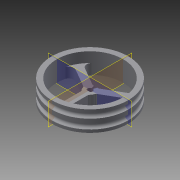
# Autodesk Inventor part: Rueda1
Saved by Autodesk Inventor 2013 (Build 170138000, 138)
## iProperties
Created: 2012-12-03
Part Number: Rueda1
Material: Generic
Document SubType Name: Modeling
Designer: ALUMNO
Density: 1 g/cm^3
Author: ALUMNO
Autodesk Inventor part; units mm, degrees
ref_plane "XY Plane" through (0, 0, 0) normal (0, 0, 1) x (1, 0, 0)
sketch "Sketch1" plane through (0, 0, 0) normal (0, 0, 1) x (1, 0, 0)
  line L0 (-19.5, 0) -> (19.5, 0) construction
  line L1 (-1.118, -1) -> (1.118, -1)
  line L2 (0, -3.5) -> (0, -10.5) construction
  line L3 (0, 31.6864) -> (0, -32.6182) construction
  line L4 (2, -2.8723) -> (2, -19.3972)
  line L5 (-2, -2.8723) -> (-2, -19.3972)
  line L6 (3.0311, 1.75) -> (9.0933, 5.25) construction
  line L7 (-3.0311, 1.75) -> (-9.0933, 5.25) construction
  line L8 (3.4875, -0.2959) -> (17.7984, 7.9665)
  line L9 (1.4875, 3.1682) -> (15.7984, 11.4306)
  arc A0 (2, -19.3972) -> (17.7984, 7.9665) centre (0, 0) ccw
  line L10 (-15.7984, 11.4306) -> (-1.4875, 3.1682)
  line L11 (-17.7984, 7.9665) -> (-3.4875, -0.2959)
  arc A1 (15.7984, 11.4306) -> (-15.7984, 11.4306) centre (0, 0) ccw
  arc A2 (-17.7984, 7.9665) -> (-2, -19.3972) centre (0, 0) ccw
  arc A3 (-3.4875, -0.2959) -> (-2, -2.8723) centre (0, 0) ccw
  arc A4 (2, -2.8723) -> (3.4875, -0.2959) centre (0, 0) ccw
  line L12 (0, 0) -> (2.0417, 7.6198) construction
  line L13 (0, 0) -> (-1.8775, 7.0067) construction
  line L14 (0.3882, 1.4489) -> (0.9059, 3.3807)
  line L15 (-0.3882, 1.4489) -> (-0.9059, 3.3807)
  arc A5 (1.4875, 3.1682) -> (0.9059, 3.3807) centre (0, 0) ccw
  arc A6 (-0.9059, 3.3807) -> (-1.4875, 3.1682) centre (0, 0) ccw
  arc A7 (1.118, -1) -> (0.3882, 1.4489) centre (0, 0) ccw
  arc A8 (-0.3882, 1.4489) -> (-1.118, -1) centre (0, 0) ccw
  circle A9 centre (0, 0) radius 22.5
  dimension "d3" = 1
  dimension "d4" = 2
  dimension "d5" = 2
  dimension "d8" = 360
  dimension "d10" = 2
  dimension "d11" = 2
  dimension "d12" = 2
  dimension "d13" = 2
  dimension "d17" = 3.5
  dimension "d18" = 3.5
  dimension "d19" = 15
  dimension "d20" = 15
  dimension "d21" = 3.5
  dimension "d22" = 3.5
  dimension "d23" = 1.5
  dimension "d24" = 1.5
  dimension "d25" = 45
  dimension "d81" = 3
  dimension "d84" = 3
  dimension "d85" = 3
  constraints: 30 end point, 21 point on circle, 10 centre point, 7 parallel, 5 point on line, 4 coincident, 1 collinear, 1 horizontal, 1 midpoint, 1 perpendicular, 10 other
  measures "d3" distance between parallel lines of L1 L0
  measures "d4" distance between parallel lines of L4 L2
  measures "d5" distance between parallel lines of L2 L5
  measures "d10" distance between parallel lines of L9 L6
  measures "d11" distance between parallel lines of L8 L6
  measures "d12" distance between parallel lines of L10 L7
  measures "d13" distance between parallel lines of L7 L11
  measures "d17" radius of A4
  measures "d18" radius of A3
  measures "d19" angle of L3 L12
  measures "d20" angle of L3 L13
  measures "d21" radius of A5
  measures "d22" radius of A6
  measures "d23" radius of A8
  measures "d24" radius of A7
  measures "d25" diameter of A9
  measures "d81" radial gap between concentric circles of A9 A1
  measures "d84" radial gap between concentric circles of A0 A9
  measures "d85" radial gap between concentric circles of A9 A2
extrude "Extrusion1" add sketch "Sketch1" along normal blind 6
fillet "Fillet10" radius 1 6 edges at (3.4875, -0.2959, 3) (2, -2.8723, 3) (-3.4875, -0.2959, 3) (-2, -2.8723, 3) (-1.4875, 3.1682, 3) (1.4875, 3.1682, 3)
fillet "Fillet11" radius 3 6 edges at (-17.7984, 7.9665, 3) (-15.7984, 11.4306, 3) (15.7984, 11.4306, 3) (17.7984, 7.9665, 3) (2, -19.3972, 3) (-2, -19.3972, 3)
sketch "Sketch5" plane through (0, 0, 6) normal (0, 0, 1) x (1, 0, 0)
  arc A0 (-19.048, 4.1741) -> (-5.9091, -18.5831) centre (0, 0) ccw projected
  circle A1 centre (0, 0) radius 22.5 projected
  circle A2 centre (0, 0) radius 22.5
  circle A3 centre (0, 0) radius 19.5
  constraints: 2 centre point, 2 coincident, 2 concentric
extrude "Extrusion2" add sketch "Sketch5" along normal blind 6
sketch "Sketch4" plane through (0, 0, 0) normal (0, 1, 0) x (-1, 0, 0)
  circle A0 centre (22.26, 3.2046) radius 1.5
  line L0 (0, 7.6708) -> (0, -6.5685) construction
  line L1 (22.4632, 5.9906) -> (22.4632, 0) construction
  circle A1 centre (22.26, 8.7046) radius 1.5
  point P0 (0, 0)
  dimension "d100" = 5.5
  constraints: 4 end point, 2 centre point, 2 vertical, 1 parallel, 2 other
  measures "d100" distance of A0.centre A1.centre
revolve "Revolution2" cut sketch "Sketch4" angle 360 about axis through (0, 0, 7.6708) along (0, 0, -1)
equation "\"d5\" = d4"
equation "\"d11\" = d10"
equation "\"d12\" = d10"
equation "\"d13\" = d10"
equation "\"d18\" = d17"
equation "\"d20\" = d19"
equation "\"d21\" = d17"
equation "\"d22\" = d17"
equation "\"d24\" = d23"
body "Solid1"
